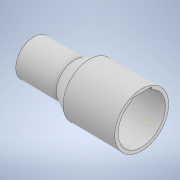
# Autodesk Inventor part: fitting non rebreathing valve v2
Saved by Autodesk Inventor 2020 (Build 240168000, 168)
## iProperties
Created: 2020-04-13
Part Number: fitting non rebreathing valve v2
Material: Generic
Document SubType Name: Modeling
Designer: Ben
Density: 1 g/cm^3
Appearance: Default
Author: Ben
Autodesk Inventor part; units mm, degrees
ref_plane "XZ Plane" through (0, 0, 0) normal (0, 1, 0) x (-1, 0, 0)
ref_plane "XY Plane" through (0, 0, 0) normal (0, 0, 1) x (1, 0, 0)
sketch "Sketch1" plane through (0, 0, 0) normal (0, 0, 1) x (1, 0, 0)
  line L0 (0.2085, 0) -> (9, 0)
  line L1 (2.2118, 14.0222) -> (2.2118, 13.8222)
  line L2 (2.2118, 13.8222) -> (5.2118, 13.8222)
  line L3 (5.2118, 13.8222) -> (5.2118, 14.0222)
  line L4 (0.2118, 14) -> (2.2118, 14.0222)
  line L5 (5.2118, 14.0222) -> (32.2118, 14.5)
  line L6 (-8.963, 9) -> (0.2118, 14)
  line L7 (-8.963, 9) -> (-33.963, 9)
  line L8 (-33.963, 9) -> (-33.963, 11)
  line L9 (-33.963, 11) -> (-8.963, 11.25)
  line L10 (-8.963, 11.25) -> (0.2118, 16.2105)
  line L11 (0.2118, 16.2105) -> (32.1937, 16.5)
  line L12 (32.1937, 16.5) -> (32.2118, 14.5)
  point P0 (0, 0)
  dimension "d1" = 14.5
  dimension "d2" = 14
  dimension "d5" = 32
  dimension "d7" = 3
  dimension "d8" = 2
  dimension "d9" = 0.2
  dimension "d10" = 0.2
  dimension "d11" = 9
  dimension "d12" = 0
  dimension "d16" = 0
  dimension "d17" = 25
  dimension "d18" = 11.25
  dimension "d19" = 11
  dimension "d20" = 0
  dimension "d21" = 2
  dimension "d23" = 25
  constraints: 26 end point, 3 perpendicular, 2 vertical, 1 horizontal
  measures "d1" vertical distance of L5.end point (0, 0)
  measures "d2" vertical distance of point (0, 0) L4.start
  measures "d5" horizontal distance of L5.end L4.start
  measures "d7" distance of L1.end L2.end
  measures "d8" horizontal distance of L4.start L1.start
  measures "d9" distance of L1.start L1.end
  measures "d10" distance of L3.end L2.end
  measures "d11" vertical distance of L0.start L6.start
  measures "d12" distance from line of point (0, 0) L0
  measures "d16" vertical distance of L6.start L7.end
  measures "d17" distance of L6.start L7.end
  measures "d18" vertical distance of L0.start L9.end
  measures "d19" vertical distance of point (0, 0) L8.end
  measures "d20" horizontal distance of L4.start L10.end
  measures "d21" vertical distance of L11.end L5.end
  measures "d23" horizontal distance of L9.end L8.end
revolve "Revolution1" add sketch "Sketch1" angle 360 about axis through (0.2085, 0, 0) along (1, 0, 0)
ref_plane "Work Plane1" through (35, 0, 0) normal (1, 0, 0) x (0, 1, 0)
sketch "Sketch2" plane through (35, 0, 0) normal (1, 0, 0) x (0, 1, 0)
  circle A0 centre (0, 0) radius 16.5 projected
  circle A1 centre (0, 0) radius 14.5 projected
  line L0 (11.5082, -6) -> (14.5, -6)
  line L1 (14.5, -6) -> (14.5, 6)
  line L2 (14.5, 6) -> (11.5082, 6)
  line L3 (11.5082, 6) -> (11.5082, -6)
  line L4 (14.695, 6) -> (14.695, -6)
  line L5 (14.695, -6) -> (14.5, -6)
  line L6 (14.695, 6) -> (14.5, 6)
  dimension "d25" = 12
  dimension "d26" = 6
  constraints: 14 end point, 3 parallel, 2 perpendicular, 1 collinear, 1 horizontal, 1 tangent
  measures "d25" distance of L2.end L0.start
  measures "d26" distance from line of point (0, 0) L0
extrude "Extrusion1" cut sketch "Sketch2" against normal blind 6.788 contours A1 L0 L3 L2 | L1 L0 A1 | A1 L2 L1 picked at (12.5055, 0)
sketch "Sketch3" plane through (35, 0, 0) normal (1, 0, 0) x (0, 1, 0)
  point P0 (0, 0)
ref_plane "Work Plane2" through (32.194, 0, 0) normal (1, 0, 0) x (0, 1, 0)
equation "\"d10\" = d9"
body "Solid1"
